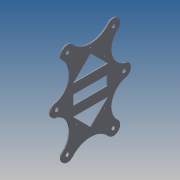
# Autodesk Inventor part: BaseBawah
Saved by Autodesk Inventor 2014 (Build 180170000, 170)
## iProperties
Created: 2014-12-20
Part Number: BaseBawah
Material: Generic
Document SubType Name: Modeling
Designer: I Was ME
Density: 1 g/cm^3
Appearance: Default
Author: I Was ME
Autodesk Inventor part; units mm, degrees
ref_plane "YZ Plane" through (0, 0, 0) normal (1, 0, 0) x (0, 1, 0)
ref_plane "XZ Plane" through (0, 0, 0) normal (0, 1, 0) x (-1, 0, 0)
ref_plane "XY Plane" through (0, 0, 0) normal (0, 0, 1) x (1, 0, 0)
sketch "Sketch1" plane through (0, 0, 0) normal (1, 0, 0) x (0, 1, 0)
  line L0 (-42.75, 165) -> (42.75, 165) construction
  line L1 (42.75, 165) -> (42.75, 0) construction
  line L2 (42.75, 0) -> (-42.75, 0) construction
  line L3 (-42.75, 0) -> (-42.75, 165) construction
  arc A0 (-32.6897, 172.419) -> (-50.4192, 155.1291) centre (-42.75, 165) ccw
  arc A1 (50.4158, 155.1265) -> (32.6897, 172.419) centre (42.75, 165) ccw
  arc A2 (-50.4296, 9.8627) -> (-32.6897, -7.419) centre (-42.75, 0) ccw
  arc A3 (32.6897, -7.419) -> (50.433, 9.8601) centre (42.75, 0) ccw
  line L4 (0, 0) -> (0, 165) construction
  line L5 (-19.1029, 0) -> (-19.1029, 82.5) construction
  line L6 (-42.75, 82.5346) -> (42.75, 82.5346) construction
  line L7 (-42.75, 82.5346) -> (-62.75, 82.5346) construction
  line L8 (42.75, 82.5346) -> (62.75, 82.5346) construction
  arc A4 (-62.75, 95.0346) -> (-62.75, 70.0346) centre (-62.75, 82.5346) ccw
  arc A5 (62.7626, 70.0346) -> (62.7374, 95.0346) centre (62.75, 82.5346) ccw
  circle A6 centre (-62.75, 82.5346) radius 3.5
  circle A7 centre (62.75, 82.5346) radius 3.5
  circle A8 centre (-42.75, 165) radius 3.5
  circle A9 centre (42.75, 165) radius 3.5
  circle A10 centre (-42.75, 0) radius 3.5
  circle A11 centre (42.75, 0) radius 3.5
  line L9 (42.75, 165) -> (33.9112, 173.8388) construction
  line L10 (-42.75, 165) -> (-33.9112, 173.8388) construction
  line L11 (42.75, 165) -> (51.5888, 156.1612) construction
  line L12 (-42.75, 165) -> (-51.5888, 156.1612) construction
  line L13 (-42.75, 0) -> (-51.5888, 8.8388) construction
  line L14 (-42.75, 0) -> (-33.9112, -8.8388) construction
  line L15 (42.75, 0) -> (33.9112, -8.8388) construction
  line L16 (42.75, 0) -> (51.5888, 8.8388) construction
  line L17 (-62.75, 82.5346) -> (-62.75, 95.0346) construction
  line L18 (-62.75, 82.5346) -> (-62.75, 70.0346) construction
  line L19 (62.75, 82.5346) -> (62.7374, 95.0346) construction
  line L20 (62.75, 82.5346) -> (62.7626, 70.0346) construction
  line L21 (-51.5888, 156.1612) -> (-62.75, 95.0346) construction
  line L22 (-33.9112, 173.8388) -> (33.9112, 173.8388) construction
  line L23 (51.5888, 156.1612) -> (62.7374, 95.0346) construction
  line L24 (62.7626, 70.0346) -> (51.5888, 8.8388) construction
  line L25 (33.9112, -8.8388) -> (-33.9112, -8.8388) construction
  line L26 (-51.5888, 8.8388) -> (-62.75, 70.0346) construction
  line L27 (-57.1694, 125.5979) -> (-39.4622, 122.3647) construction
  line L28 (57.1631, 125.5979) -> (39.4552, 122.3682) construction
  line L29 (-57.1694, 39.4367) -> (-39.4615, 42.6664) construction
  line L30 (57.1757, 39.4367) -> (39.4685, 42.6699) construction
  line L31 (0, -8.8388) -> (0, 7.1612)
  arc A12 (-33.9112, 173.8388) -> (33.9112, 173.8388) centre (0, 201.7753) ccw
  arc A13 (-62.75, 95.0346) -> (-51.5888, 156.1612) centre (-74.6924, 128.7974) ccw
  arc A14 (-51.5888, 8.8388) -> (-62.75, 70.0346) centre (-74.7509, 36.2301) ccw
  arc A15 (62.7626, 70.0346) -> (51.5888, 8.8388) centre (74.7585, 36.2263) ccw
  arc A16 (33.9112, -8.8388) -> (-33.9112, -8.8388) centre (0, -36.7753) ccw
  arc A17 (51.5888, 156.1612) -> (62.7374, 95.0346) centre (74.6848, 128.7936) ccw
  line L32 (-42.75, 99.1738) -> (-31.75, 99.1738) construction
  line L33 (42.75, 99.1738) -> (31.75, 99.1738) construction
  line L34 (0, 157.8388) -> (0, 7.1612) construction
  line L35 (-25.75, 165) -> (-25.75, 103.3033) construction
  line L36 (-31.75, 91.7175) -> (31.75, 91.7175)
  line L37 (31.75, 91.7175) -> (31.75, 73.7175)
  line L38 (31.75, 73.7175) -> (-31.75, 73.7175)
  line L39 (-31.75, 73.7175) -> (-31.75, 91.7175)
  line L40 (0, 142.2444) -> (-32.5269, 109.7175)
  line L41 (-32.5269, 109.7175) -> (32.5269, 109.7175)
  line L42 (32.5269, 109.7175) -> (0, 142.2444)
  line L43 (0, 23.1637) -> (-32.5, 55.7175)
  line L44 (-32.5, 55.7175) -> (32.5, 55.7175)
  line L45 (32.5, 55.7175) -> (0, 23.1637)
  circle A18 centre (0, 151.3388) radius 1
  circle A19 centre (25.75, 124.7175) radius 1
  circle A20 centre (-25.75, 124.7175) radius 1
  circle A21 centre (-25.75, 40.7175) radius 1
  circle A22 centre (25.75, 40.7175) radius 1
  dimension "d0" = 165
  dimension "d1" = 85.5
  dimension "d2" = 82.5
  dimension "d3" = 20
  dimension "d4" = 20
  dimension "d5" = 25
  dimension "d6" = 25
  dimension "d7" = 25
  dimension "d8" = 25
  dimension "d9" = 25
  dimension "d10" = 25
  dimension "d11" = 7
  dimension "d12" = 7
  dimension "d13" = 7
  dimension "d14" = 7
  dimension "d15" = 7
  dimension "d16" = 7
  dimension "d17" = 45
  dimension "d18" = 45
  dimension "d19" = 45
  dimension "d20" = 45
  dimension "d21" = 45
  dimension "d22" = 45
  dimension "d23" = 45
  dimension "d24" = 90
  dimension "d26" = 16
  dimension "d27" = 11
  dimension "d28" = 11
  dimension "d29" = 150.6777
  dimension "d30" = 61.6967
  dimension "d31" = 63.5
  dimension "d32" = 18
  dimension "d33" = 73.2825
  dimension "d34" = 31
  dimension "d35" = 46
  dimension "d36" = 46
  dimension "d37" = 65.0538
  dimension "d38" = 18
  dimension "d39" = 65
  dimension "d40" = 46
  dimension "d41" = 46
  dimension "d42" = 18
  dimension "d43" = 2
  dimension "d44" = 6.5
  dimension "d45" = 2
  dimension "d46" = 2
  dimension "d47" = 33
  dimension "d48" = 17
  dimension "d49" = 17
  dimension "d50" = 33
  dimension "d51" = 2
  dimension "d52" = 2
  dimension "d53" = 33
  dimension "d54" = 33
  dimension "d55" = 17
  dimension "d56" = 17
  constraints: 92 end point, 46 point on circle, 23 centre point, 13 coincident, 12 perpendicular, 12 point on line, 11 parallel, 7 midpoint, 5 collinear, 2 horizontal, 1 equal length
  measures "d0" distance of L3.start L3.end
  measures "d1" distance of L1.end L3.start
  measures "d2" distance of L5.start L5.end
  measures "d3" distance of L7.start L7.end
  measures "d4" distance of L8.start L8.end
  measures "d5" diameter of A4
  measures "d6" diameter of A5
  measures "d7" diameter of A1
  measures "d8" diameter of A0
  measures "d9" diameter of A3
  measures "d10" diameter of A2
  measures "d11" diameter of A10
  measures "d12" diameter of A11
  measures "d13" diameter of A7
  measures "d14" diameter of A6
  measures "d15" diameter of A9
  measures "d16" diameter of A8
  measures "d17" angle of L0 L9
  measures "d18" angle of L1 L11
  measures "d19" angle of L3 L12
  measures "d20" angle of L3 L13
  measures "d21" angle of L2 L14
  measures "d22" angle of L1 L16
  measures "d23" angle of L2 L15
  measures "d24" angle of L26 L29
  measures "d26" distance of L31.start L34.end
  measures "d27" distance of L32.start L32.end
  measures "d28" distance of L33.start L33.end
  measures "d29" distance of L34.start L34.end
  measures "d30" distance of L35.start L35.end
  measures "d31" distance of L39.end L36.end
  measures "d32" distance of L39.start L39.end
  measures "d33" distance between parallel lines of L36 L0
  measures "d34" distance from line of L7.end L39
  measures "d35" distance of L40.start L40.end
  measures "d36" distance of L42.start L40.start
  measures "d37" distance of L40.end L42.start
  measures "d38" distance between parallel lines of L36 L41
  measures "d39" distance of L44.start L45.start
  measures "d40" distance of L45.end L44.start
  measures "d41" distance of L45.start L45.end
  measures "d42" distance between parallel lines of L38 L44
  measures "d43" diameter of A18
  measures "d44" distance of A18.centre L34.start
  measures "d45" diameter of A19
  measures "d46" diameter of A20
  measures "d47" distance from line of L36 A19.centre
  measures "d48" distance from line of L1 A19.centre
  measures "d49" distance from line of L3 A20.centre
  measures "d50" distance from line of L36 A20.centre
  measures "d51" diameter of A22
  measures "d52" diameter of A21
  measures "d53" distance from line of L38 A21.centre
  measures "d54" distance from line of L38 A22.centre
  measures "d55" distance from line of L3 A21.centre
  measures "d56" distance from line of L1 A22.centre
extrude "Extrusion1" add sketch "Sketch1" along normal blind 2 contours A12 A1 A17 A5 A15 A3 A16 A2 A14 A4 A13 A0
body "Solid1"
